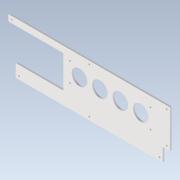
# Autodesk Inventor part: BasePlate
Saved by Autodesk Inventor 2022.2 (Build 262287000, 287)
## iProperties
Created: 2021-12-01
Part Number: BasePlate
Material: Generic
Document SubType Name: Modeling
Designer: Fabijan_Sven
Density: 1 g/cm^3
Appearance: Default
Author: Fabijan_Sven
Autodesk Inventor part; units mm, degrees
ref_plane "YZ Plane" through (0, 0, 0) normal (1, 0, 0) x (0, 1, 0)
ref_plane "XZ Plane" through (0, 0, 0) normal (0, 1, 0) x (-1, 0, 0)
ref_plane "XY Plane" through (0, 0, 0) normal (0, 0, 1) x (1, 0, 0)
sketch "Sketch1" plane through (0, 0, 0) normal (0, 0, 1) x (1, 0, 0)
  line L0 (500, 160) -> (0, 160)
  line L1 (0, 160) -> (0, 140)
  line L2 (478, 0) -> (478, 42)
  line L3 (478, 42) -> (500, 42)
  line L4 (500, 42) -> (500, 160)
  line L5 (0, 0) -> (22, 0)
  line L6 (22, 0) -> (22, 40)
  line L7 (22, 0) -> (478, 0)
  line L8 (0, 42) -> (0, 0)
  line L9 (0, 140) -> (170, 140)
  line L10 (170, 140) -> (170, 40)
  line L11 (170, 40) -> (22, 40)
  line L12 (0, 56) -> (0, 42)
  dimension "d1" = 500
  dimension "d6" = 22
  dimension "d46" = 42
  dimension "d47" = 160
  dimension "d52" = 20
  dimension "d53" = 170
  dimension "d54" = 40
  constraints: 26 end point, 5 parallel, 3 horizontal, 3 perpendicular, 1 collinear
  measures "d1" distance of L0.start L0.end
  measures "d6" distance between parallel lines of L4 L2
  measures "d46" distance of L2.start L2.end
  measures "d47" distance between parallel lines of L7 L0
  measures "d52" distance between parallel lines of L9 L0
  measures "d53" distance between parallel lines of L10 L1
  measures "d54" distance between parallel lines of L11 L7
extrude "Extrusion1" add sketch "Sketch1" along normal blind 5
sketch "Sketch2" plane through (0, 0, 5) normal (0, 0, 1) x (1, 0, 0)
  circle A0 centre (32, 10) radius 2.75
  circle A1 centre (468, 10) radius 2.75
  circle A2 centre (10, 150) radius 2.75
  circle A3 centre (490, 150) radius 2.75
  circle A4 centre (490, 52) radius 2.75
  line L0 (500, 160) -> (0, 160) projected
  line L1 (500, 42) -> (500, 160) projected
  line L2 (478, 42) -> (500, 42) projected
  line L3 (478, 0) -> (478, 42) projected
  circle A5 centre (190, 130) radius 3.25
  circle A6 centre (440, 130) radius 3.25
  circle A7 centre (190, 70) radius 3.25
  circle A8 centre (440, 70) radius 3.25
  line L4 (0, 160) -> (0, 140) projected
  line L5 (22, 0) -> (478, 0) projected
  line L6 (22, 40) -> (22, 0) projected
  circle A9 centre (250, 150) radius 2.75
  circle A10 centre (250, 10) radius 2.75
  dimension "d9" = 5.5
  dimension "d10" = 10
  dimension "d12" = 10
  dimension "d13" = 10
  dimension "d14" = 10
  dimension "d15" = 10
  dimension "d16" = 10
  dimension "d20" = 5.5
  dimension "d21" = 5.5
  dimension "d22" = 5.5
  dimension "d23" = 5.5
  dimension "d34" = 60
  dimension "d35" = 60
  dimension "d38" = 30
  dimension "d39" = 6.5
  dimension "d40" = 6.5
  dimension "d41" = 6.5
  dimension "d42" = 6.5
  dimension "d43" = 30
  dimension "d55" = 70
  dimension "d56" = 190
  dimension "d57" = 190
  dimension "d58" = 10
  dimension "d59" = 10
  dimension "d60" = 10
  dimension "d61" = 10
  dimension "d62" = 70
  dimension "d63" = 10
  dimension "d64" = 10
  dimension "d65" = 5.5
  dimension "d66" = 5.5
  dimension "d67" = 250
  dimension "d68" = 250
  constraints: 11 centre point
  measures "d9" diameter of A2
  measures "d10" distance from line of L0 A2.centre
  measures "d12" distance from line of A3.centre L0
  measures "d13" distance from line of L1 A3.centre
  measures "d14" distance from line of A4.centre L1
  measures "d15" distance from line of L2 A4.centre
  measures "d16" distance from line of L3 A1.centre
  measures "d20" diameter of A3
  measures "d21" diameter of A4
  measures "d22" diameter of A1
  measures "d23" diameter of A0
  measures "d34" distance from line of L1 A6.centre
  measures "d35" distance from line of L1 A8.centre
  measures "d38" distance from line of L0 A5.centre
  measures "d39" diameter of A5
  measures "d40" diameter of A6
  measures "d41" diameter of A8
  measures "d42" diameter of A7
  measures "d43" distance from line of L0 A6.centre
  measures "d55" distance from line of L5 A7.centre
  measures "d56" distance from line of L4 A5.centre
  measures "d57" distance from line of L4 A7.centre
  measures "d58" distance from line of L6 A0.centre
  measures "d59" distance from line of L4 A2.centre
  measures "d60" distance from line of L5 A0.centre
  measures "d61" distance from line of L5 A1.centre
  measures "d62" distance from line of L5 A8.centre
  measures "d63" distance from line of L0 A9.centre
  measures "d64" distance from line of L5 A10.centre
  measures "d65" diameter of A9
  measures "d66" diameter of A10
  measures "d67" distance from line of A9.centre L1
  measures "d68" distance from line of A10.centre L1
fillet "Fillet1" radius 2 9 edges at (500, 160, 2.5) (500, 42, 2.5) (0, 160, 2.5) (478, 0, 2.5) (22, 0, 2.5) (22, 40, 2.5) (0, 140, 2.5) (170, 140, 2.5) (170, 40, 2.5)
hole "Hole6" at (10, 150, 5) at (250, 150, 5) at (490, 150, 5) at (490, 52, 5) at (468, 10, 5) at (250, 10, 5) at (32, 10, 5) at (190, 130, 5) at (190, 70, 5) at (440, 130, 5) at (440, 70, 5) direction (0, 0, -1) diameter 5.5 end through all
sketch "Sketch4" plane through (0, 0, 5) normal (0, 0, 1) x (1, 0, 0)
  circle A0 centre (220, 100) radius 24
  circle A1 centre (283.3333, 100) radius 24
  circle A2 centre (346.6667, 100) radius 24
  circle A3 centre (410, 100) radius 24
  circle A4 centre (190, 130) radius 2.75 projected
  line L0 (207.2246, 100) -> (486.1087, 100) construction
  point P0 (0, 0)
  dimension "d115" = 30
  dimension "d116" = 30
  dimension "d117" = 63.3333
  dimension "d118" = 63.3333
  dimension "d119" = 63.3333
  dimension "d120" = 48
  dimension "d121" = 48
  dimension "d122" = 48
  dimension "d123" = 48
  constraints: 4 centre point, 3 point on line, 2 end point, 1 coincident, 1 horizontal, 1 midpoint
  measures "d115" distance from line of L0 A4.centre
  measures "d116" horizontal distance of A0.centre A4.centre
  measures "d117" distance of A1.centre A0.centre
  measures "d118" distance of A2.centre A1.centre
  measures "d119" distance of A3.centre A2.centre
  measures "d120" diameter of A0
  measures "d121" diameter of A1
  measures "d122" diameter of A2
  measures "d123" diameter of A3
extrude "Extrusion2" cut sketch "Sketch4" against normal blind 10 contours A0 | A1 | A2 | A3
equation "\"d12\" = d10"
equation "\"d13\" = d10"
equation "\"d14\" = d10"
equation "\"d15\" = d10"
equation "\"d16\" = d10"
equation "\"d20\" = d9"
equation "\"d21\" = d9"
equation "\"d22\" = d9"
equation "\"d23\" = d9"
equation "\"d35\" = d34"
equation "\"d40\" = d39"
equation "\"d41\" = d39"
equation "\"d42\" = d39"
equation "\"d43\" = d38"
equation "\"d57\" = d56"
equation "\"d58\" = d10"
equation "\"d59\" = d10"
equation "\"d60\" = d10"
equation "\"d61\" = d10"
equation "\"d62\" = d55"
equation "\"d63\" = d10"
equation "\"d64\" = d10"
equation "\"d65\" = d9"
equation "\"d66\" = d9"
equation "\"d68\" = d67"
equation "\"d97\" = d9"
equation "\"d118\" = d117"
equation "\"d119\" = d117"
equation "\"d121\" = d120"
equation "\"d122\" = d120"
equation "\"d123\" = d120"
body "Solid1"
